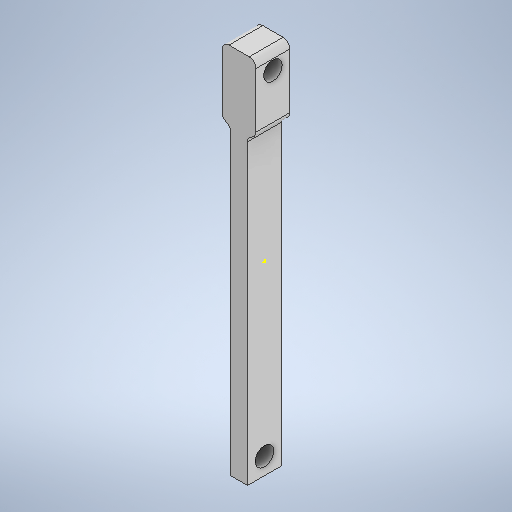
# Autodesk Inventor part: element_posredni
Saved by Autodesk Inventor 2025.2 (Build 292293000, 293)
## iProperties
Created: 2025-11-26
Part Number: element_posredni
Material: Ogólny
Document SubType Name: Modeling
Designer: juras
Density: 1 g/cm^3
Appearance: Domyślna
Author: juras
Autodesk Inventor part; units mm, degrees
ref_plane "YZ Plane" through (0, 0, 0) normal (1, 0, 0) x (0, 1, 0)
ref_plane "XZ Plane" through (0, 0, 0) normal (0, 1, 0) x (-1, 0, 0)
ref_plane "XY Plane" through (0, 0, 0) normal (0, 0, 1) x (1, 0, 0)
sketch "Szkic1" plane through (0, 0, 0) normal (0, 1, 0) x (-1, 0, 0)
  line L0 (-2.5, -5) -> (2.5, -5)
  line L1 (2.5, -5) -> (2.5, 5)
  line L2 (2.5, 5) -> (-2.5, 5)
  line L3 (-2.5, 5) -> (-2.5, -5)
  line L4 (-2.5, -5) -> (2.5, 5) construction
  line L5 (2.5, -5) -> (-2.5, 5) construction
  point P0 (0, 0)
  dimension "d0" = 5
  dimension "d1" = 10
  constraints: 12 end point, 2 midpoint, 2 parallel, 1 horizontal, 1 perpendicular
  measures "d0" distance of L2.end L1.end
  measures "d1" distance of L1.end L0.end
extrude "Wyciągnięcie proste1" add sketch "Szkic1" along normal mid plane 110
sketch "Szkic3" plane through (2.5, -55, 5) normal (1, 0, 0) x (0, 0, -1)
  circle A0 centre (5, 5) radius 2.75
  line L0 (10, 0) -> (0, 0) projected
  line L1 (10, 0) -> (10, 110) projected
  point P0 (5, 55)
  point P1 (10, 118)
  dimension "d10" = 5.5
  dimension "d11" = 5
  dimension "d12" = 5
  constraints: 1 centre point
  measures "d10" diameter of A0
  measures "d11" distance from line of L0 A0.centre
  measures "d12" distance from line of L1 A0.centre
extrude "Wyciągnięcie proste3" cut sketch "Szkic3" against normal blind 120
sketch "Szkic4" plane through (2.5, -55, -5) normal (1, 0, 0) x (0, 0, -1)
  point P0 (-5, 55)
sketch "Szkic5" plane through (0, 55, 0) normal (0, 1, 0) x (1, 0, 0)
  line L0 (5, -5) -> (-5, -5)
  line L1 (-5, -5) -> (-5, 5)
  line L2 (-5, 5) -> (5, 5)
  line L3 (5, 5) -> (5, -5)
  line L4 (5, -5) -> (-5, 5) construction
  line L5 (-5, -5) -> (5, 5) construction
  point P0 (0, 0)
  dimension "d16" = 10
  dimension "d17" = 10
  constraints: 12 end point, 2 midpoint, 2 parallel, 1 horizontal, 1 perpendicular
  measures "d16" distance of L1.end L2.end
  measures "d17" distance of L0.end L1.end
extrude "Wyciągnięcie proste4" add sketch "Szkic5" against normal blind 20
sketch "Szkic6" plane through (5, 55, 5) normal (1, 0, 0) x (0, 0, -1)
  circle A0 centre (5, -5) radius 2.75
  line L0 (0, 0) -> (10, 0) projected
  line L1 (0, 0) -> (0, -20) projected
  point P0 (5, -55)
  dimension "d20" = 5.5
  dimension "d21" = 5
  dimension "d22" = 5
  constraints: 1 centre point
  measures "d20" diameter of A0
  measures "d21" distance from line of A0.centre L0
  measures "d22" distance from line of A0.centre L1
extrude "Wyciągnięcie proste5" cut sketch "Szkic6" against normal blind 20
fillet "Zaokrąglenie3" radius 2 6 edges at (2.5, 35, 0) (5, 35, 0) (-5, 35, 0) (-2.5, 35, 0) (-5, 55, 0) (5, 55, 0)
